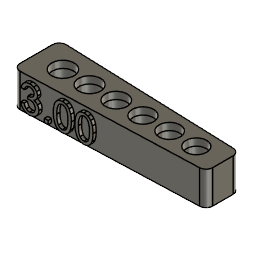
HoleDiaTest3mm_v1 (Autodesk Fusion 360 design; units mm, degrees)
Autodesk Fusion 360 part; units mm, degrees
sketch "Sketch1" plane through (0, 0, 0) normal (0, 0, 1) x (1, 0, 0)
  circle A0 centre (0, 0) radius 1.5
  circle A1 centre (4, 0) radius 1.475
  circle A2 centre (8, 0) radius 1.45
  circle A3 centre (-4, 0) radius 1.525
  circle A4 centre (-8, 0) radius 1.55
  circle A5 centre (-12, 0) radius 1.575
  line L0 (-12, 0) -> (8, 0) construction
  line L1 (8, 0) -> (7.5, 0) construction
  line L2 (-12, 0) -> (-16, 0) construction
  line L3 (8, 0) -> (12, 0) construction
  line L4 (-16, -3.5) -> (-16, 3.5)
  line L5 (12, -2.5) -> (12, 2.5)
  line L6 (12, 2.5) -> (-16, 3.5)
  line L7 (-16, -3.5) -> (12, -2.5)
  dimension "d1" = 3
  dimension "d2" = 2.95
  dimension "d3" = 2.9
  dimension "d4" = 3.05
  dimension "d5" = 3.1
  dimension "d6" = 3.15
  dimension "d7" = 4
  dimension "d8" = 4
  dimension "d10" = 4
  dimension "d11" = 4
  dimension "d25" = 4
  dimension "d29" = 4
  dimension "d30" = 4
  constraint coincident A5.centre L0.start
  constraint coincident A2.centre L0.end
  constraint parallel L0 L1
  constraint parallel L0 L2
  constraint parallel L0 L3
  constraint midpoint L2.end L4
  constraint perpendicular L2 L4
  constraint midpoint L3.end L5
  constraint perpendicular L3 L5
  measures "d1" diameter of A0
  measures "d2" diameter of A1
  measures "d3" diameter of A2
  measures "d4" diameter of A3
  measures "d5" diameter of A4
  measures "d6" diameter of A5
  measures "d7" distance of A4.centre A5.centre
  measures "d8" distance of A3.centre A4.centre
  measures "d10" distance of A0.centre A1.centre
  measures "d11" distance of A1.centre A2.centre
  measures "d25" distance of A0.centre A3.centre
  measures "d29" distance of A5.centre L2.end
  measures "d30" distance of A2.centre L3.end
extrude "Extrude1" add sketch "Sketch1" against normal blind 5
fillet "Fillet2" radius 1 4 edges at (-16, 3.5, -2.5) (-16, -3.5, -2.5) (12, 2.5, -2.5) (12, -2.5, -2.5)
chamfer "Chamfer2" distance 0.1 distance2 1 6 edges at (-13.4684, -0.5695, -5) (-9.4451, -0.5605, -5) (-5.4218, -0.5515, -5) (-1.3985, -0.5424, -5) (2.6248, -0.5334, -5) (6.6481, -0.5243, -5) measured on face at (-15.1917, 0, -5) measured on face at (-15.1917, 0, -5) measured on face at (-15.1917, 0, -5) measured on face at (-15.1917, 0, -5) measured on face at (-15.1917, 0, -5) measured on face at (-15.1917, 0, -5) tangent chain off
chamfer "Chamfer3" distance 1 distance2 0.1 6 edges at (-13.4684, -0.5695, 0) (-9.4451, -0.5605, 0) (-5.4218, -0.5515, 0) (-1.3985, -0.5424, 0) (2.6248, -0.5334, 0) (6.6481, -0.5243, 0) measured on face at (-10.427, -0.0785, -2.6667) measured on face at (-6.4519, -0.0773, -2.6667) measured on face at (-2.4769, -0.076, -2.6667) measured on face at (1.4981, -0.0748, -2.6667) measured on face at (5.4732, -0.0735, -2.6667) measured on face at (9.4482, -0.0723, -2.6667) tangent chain off
sketch "Sketch2" plane through (0.1045, -2.9248, 0) normal (0.035692, -0.999363, 0) x (0.999363, 0.035692, 0)
  line L0 (10.9382, -5) -> (10.9382, 0)
  line L1 (10.9382, 0) -> (-15.0784, 0)
  line L2 (-15.0784, 0) -> (-15.0784, -5)
  line L3 (-15.0784, -5) -> (10.9382, -5)
  line L4 (-14.5, -4.5) -> (7.5, -4.5) construction
  line L5 (7.5, -4.5) -> (7.5, -0.5) construction
  line L6 (7.5, -0.5) -> (-14.5, -0.5) construction
  line L7 (-14.5, -0.5) -> (-14.5, -4.5) construction
  dimension "d37" = 4
  dimension "d38" = 0
  text T0 "3.00" font "Arial" height 4 align left top in box 22 x 4 at (-14.5, -4.5) x (1, 0) y (0, 1) spacing 1.01 kerned
extrude "Extrude3" add sketch "Sketch2" along normal blind 0.5 text T0
equation "d38 = '3.00'"
